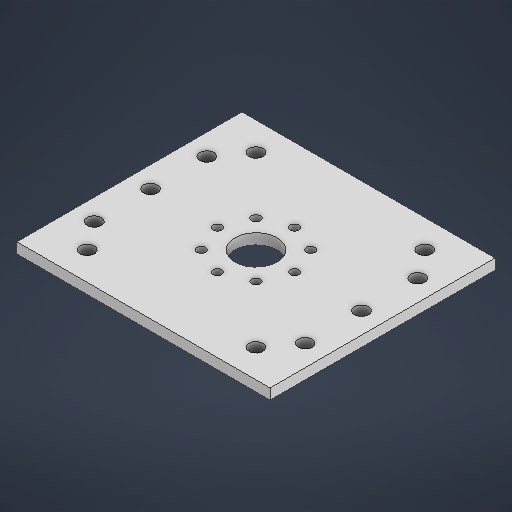
# Autodesk Inventor part: FifthAxisServoPlate
Saved by Autodesk Inventor 2025 (Build 290162000, 162)
## iProperties
Created: 2024-05-20
Part Number: FifthAxisServoPlate
Material: Generic
Document SubType Name: Modeling
Designer: avsar
Density: 1 g/cm^3
Appearance: Default
Author: avsar
Autodesk Inventor part; units mm, degrees
ref_plane "YZ Plane" through (0, 0, 0) normal (1, 0, 0) x (0, 1, 0)
ref_plane "XZ Plane" through (0, 0, 0) normal (0, 1, 0) x (-1, 0, 0)
ref_plane "XY Plane" through (0, 0, 0) normal (0, 0, 1) x (1, 0, 0)
sketch "Sketch1" plane through (0, 0, 0) normal (0, 1, 0) x (-1, 0, 0)
  line L0 (36, 32) -> (-36, 32)
  line L1 (-36, 32) -> (-36, -32)
  line L2 (-36, -32) -> (36, -32)
  line L3 (36, -32) -> (36, 32)
  line L4 (36, 32) -> (-36, -32) construction
  line L5 (-36, 32) -> (36, -32) construction
  circle A0 centre (0, 0) radius 6
  circle A1 centre (0, -11) radius 1.25
  circle A2 centre (7.7782, -7.7782) radius 1.25
  circle A3 centre (11, 0) radius 1.25
  circle A4 centre (7.7782, 7.7782) radius 1.25
  circle A5 centre (0, 11) radius 1.25
  circle A6 centre (-7.7782, 7.7782) radius 1.25
  circle A7 centre (-11, 0) radius 1.25
  circle A8 centre (-7.7782, -7.7782) radius 1.25
  circle A9 centre (24, -24) radius 2
  line L6 (0, 0) -> (0, 6) construction
  circle A10 centre (-24, -24) radius 2
  line L7 (0, 0) -> (-36, 0) construction
  circle A11 centre (24, 24) radius 2
  circle A12 centre (-24, 24) radius 2
  circle A13 centre (30, 16) radius 2
  circle A14 centre (-30, 16) radius 2
  circle A15 centre (30, -16) radius 2
  circle A16 centre (-30, -16) radius 2
  circle A17 centre (-30, 0) radius 2
  circle A18 centre (30, 0) radius 2
  dimension "d2" = 12
  dimension "d0" = 72
  dimension "d1" = 64
  dimension "d3" = 2.5
  dimension "d4" = 11
  dimension "d7" = 360
  dimension "d9" = 4
  dimension "d10" = 24
  dimension "d11" = 24
  dimension "d14" = 4
  dimension "d15" = 6
  dimension "d16" = 8
  dimension "d17" = 4
  dimension "d18" = 4
  constraints: 18 centre point, 16 end point, 6 symmetric about line, 4 vertical alignment, 3 midpoint, 2 parallel, 2 point on line, 1 coincident, 1 horizontal, 1 perpendicular, 1 vertical, 25 other
  measures "d0" distance of L2.end L1.end
  measures "d1" distance of L1.end L0.end
  measures "d3" diameter of A1
  measures "d4" distance of point (0, 0) A1.centre
  measures "d9" diameter of A9
  measures "d10" horizontal distance of A9.centre point (0, 0)
  measures "d11" horizontal distance of point (0, 0) A9.centre
  measures "d14" diameter of A13
  measures "d15" horizontal distance of A13.centre A11.centre
  measures "d16" vertical distance of A11.centre A13.centre
  measures "d17" diameter of A17
  measures "d18" diameter of A18
extrude "Extrusion1" add sketch "Sketch1" along normal blind 3
body "Solid1"
